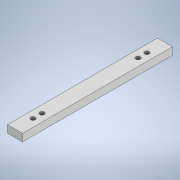
# Autodesk Inventor part: Soporte2_Dos
Saved by Autodesk Inventor 2021 (Build 250183000, 183)
## iProperties
Created: 2023-12-04
Part Number: Soporte2_Dos
Material: Generic
Document SubType Name: Modeling
Designer: Nicol
Density: 1 g/cm^3
Appearance: Default
Author: Nicol
Autodesk Inventor part; units mm, degrees
ref_plane "YZ Plane" through (0, 0, 0) normal (1, 0, 0) x (0, 1, 0)
ref_plane "XZ Plane" through (0, 0, 0) normal (0, 1, 0) x (-1, 0, 0)
ref_plane "XY Plane" through (0, 0, 0) normal (0, 0, 1) x (1, 0, 0)
sketch "Sketch1" plane through (0, 0, 0) normal (0, 1, 0) x (-1, 0, 0)
  line L0 (0, 0) -> (10, 0)
  line L1 (10, 0) -> (10, -100)
  line L2 (10, -100) -> (0, -100)
  line L3 (0, -100) -> (0, 0)
  dimension "d0" = 10
  dimension "d1" = 100
  constraints: 8 end point, 2 parallel, 1 horizontal, 1 perpendicular
  measures "d0" distance of L1.end L2.end
  measures "d1" distance of L0.end L1.end
extrude "Extrusion1" add sketch "Sketch1" along normal blind 5
sketch "Sketch2" plane through (0, 5, 0) normal (0, 1, 0) x (1, 0, 0)
  circle A0 centre (-5, 12) radius 1.5
  line L0 (0, 0) -> (0, 100) projected
  line L1 (-10, 0) -> (0, 0) projected
  circle A1 centre (-5, 18) radius 1.5
  line L2 (0, 0) -> (0, 50)
  circle A2 centre (-5, 88) radius 1.5
  circle A3 centre (-5, 82) radius 1.5
  dimension "d4" = 3
  dimension "d8" = 5
  dimension "d9" = 12
  dimension "d12" = 3
  dimension "d13" = 6
  dimension "d14" = 0
  dimension "d15" = 50
  constraints: 4 centre point, 2 end point, 1 midpoint
  measures "d4" diameter of A0
  measures "d8" distance from line of L0 A0.centre
  measures "d9" distance from line of L1 A0.centre
  measures "d12" diameter of A1
  measures "d13" distance of A1.centre A0.centre
  measures "d14" horizontal distance of A0.centre A1.centre
  measures "d15" distance of L0.start L2.end
extrude "Extrusion2" cut sketch "Sketch2" against normal through all
body "Solid1"
